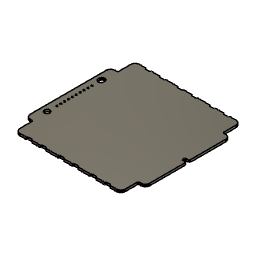
usrr5 board v2 (Autodesk Fusion 360 design; units mm, degrees)
Autodesk Fusion 360 part; units mm, degrees
sketch "Sketch1" plane through (0, 0, 0) normal (0, 1, 0) x (1, 0, 0)
  line L0 (44.246, 27.952) -> (40.2487, 27.952)
  line L1 (40.2487, 27.952) -> (40.2231, 27.9018)
  line L2 (40.2231, 27.9018) -> (40.1976, 27.8251)
  line L3 (40.1976, 27.8251) -> (40.1976, 27.774)
  line L4 (40.1976, 27.774) -> (40.1465, 27.7229)
  line L5 (40.1465, 27.7229) -> (40.1209, 27.6471)
  line L6 (40.1209, 27.6471) -> (40.0707, 27.6216)
  line L7 (40.0707, 27.6216) -> (40.0452, 27.5705)
  line L8 (40.0452, 27.5705) -> (39.9941, 27.5449)
  line L9 (39.9941, 27.5449) -> (39.9174, 27.4938)
  line L10 (39.9174, 27.4938) -> (39.8663, 27.4938)
  line L11 (39.8663, 27.4938) -> (39.7905, 27.4683)
  line L12 (39.7905, 27.4683) -> (38.1861, 27.4683)
  line L13 (38.1861, 27.4683) -> (38.1095, 27.4938)
  line L14 (38.1095, 27.4938) -> (38.0593, 27.4938)
  line L15 (38.0593, 27.4938) -> (38.0082, 27.5449)
  line L16 (38.0082, 27.5449) -> (37.9315, 27.5705)
  line L17 (37.9315, 27.5705) -> (37.906, 27.6216)
  line L18 (37.906, 27.6216) -> (37.8549, 27.6471)
  line L19 (37.8549, 27.6471) -> (37.8302, 27.6974)
  line L20 (37.8302, 27.6974) -> (37.7791, 27.774)
  line L21 (37.7791, 27.774) -> (37.7791, 27.8251)
  line L22 (37.7791, 27.8251) -> (37.7535, 27.9018)
  line L23 (37.7535, 27.9018) -> (37.728, 27.952)
  line L24 (37.728, 27.952) -> (31.9738, 27.952)
  line L25 (31.9738, 27.952) -> (31.9738, 27.9018)
  line L26 (31.9738, 27.9018) -> (31.9483, 27.8251)
  line L27 (31.9483, 27.8251) -> (31.9483, 27.774)
  line L28 (31.9483, 27.774) -> (31.8972, 27.7229)
  line L29 (31.8972, 27.7229) -> (31.8716, 27.6471)
  line L30 (31.8716, 27.6471) -> (31.8205, 27.6216)
  line L31 (31.8205, 27.6216) -> (31.7959, 27.5705)
  line L32 (31.7959, 27.5705) -> (31.7448, 27.5449)
  line L33 (31.7448, 27.5449) -> (31.6681, 27.4938)
  line L34 (31.6681, 27.4938) -> (31.617, 27.4938)
  line L35 (31.617, 27.4938) -> (31.5412, 27.4683)
  line L36 (31.5412, 27.4683) -> (29.9368, 27.4683)
  line L37 (29.9368, 27.4683) -> (29.8602, 27.4938)
  line L38 (29.8602, 27.4938) -> (29.8091, 27.4938)
  line L39 (29.8091, 27.4938) -> (29.7589, 27.5449)
  line L40 (29.7589, 27.5449) -> (29.6822, 27.5705)
  line L41 (29.6822, 27.5705) -> (29.6567, 27.6216)
  line L42 (29.6567, 27.6216) -> (29.6056, 27.6471)
  line L43 (29.6056, 27.6471) -> (29.58, 27.6974)
  line L44 (29.58, 27.6974) -> (29.5298, 27.774)
  line L45 (29.5298, 27.774) -> (29.5298, 27.8251)
  line L46 (29.5298, 27.8251) -> (29.5042, 27.9018)
  line L47 (29.5042, 27.9018) -> (29.4787, 27.952)
  line L48 (29.4787, 27.952) -> (25.4814, 27.952)
  line L49 (25.4814, 27.952) -> (25.4558, 27.9018)
  line L50 (25.4558, 27.9018) -> (25.4303, 27.8251)
  line L51 (25.4303, 27.8251) -> (25.4303, 27.774)
  line L52 (25.4303, 27.774) -> (25.3792, 27.7229)
  line L53 (25.3792, 27.7229) -> (25.3536, 27.6471)
  line L54 (25.3536, 27.6471) -> (25.3025, 27.6216)
  line L55 (25.3025, 27.6216) -> (25.2778, 27.5705)
  line L56 (25.2778, 27.5705) -> (25.2267, 27.5449)
  line L57 (25.2267, 27.5449) -> (25.1501, 27.4938)
  line L58 (25.1501, 27.4938) -> (25.099, 27.4938)
  line L59 (25.099, 27.4938) -> (25.0232, 27.4683)
  line L60 (25.0232, 27.4683) -> (23.4188, 27.4683)
  line L61 (23.4188, 27.4683) -> (23.3422, 27.4938)
  line L62 (23.3422, 27.4938) -> (23.2911, 27.4938)
  line L63 (23.2911, 27.4938) -> (23.2408, 27.5449)
  line L64 (23.2408, 27.5449) -> (23.1642, 27.5705)
  line L65 (23.1642, 27.5705) -> (23.1386, 27.6216)
  line L66 (23.1386, 27.6216) -> (23.0875, 27.6471)
  line L67 (23.0875, 27.6471) -> (23.062, 27.6974)
  line L68 (23.062, 27.6974) -> (23.0118, 27.774)
  line L69 (23.0118, 27.774) -> (23.0118, 27.8251)
  line L70 (23.0118, 27.8251) -> (22.9862, 27.9018)
  line L71 (22.9862, 27.9018) -> (22.9862, 27.952)
  line L72 (22.9862, 27.952) -> (17.2321, 27.952)
  line L73 (17.2321, 27.952) -> (17.2065, 27.9018)
  line L74 (17.2065, 27.9018) -> (17.181, 27.8251)
  line L75 (17.181, 27.8251) -> (17.181, 27.774)
  line L76 (17.181, 27.774) -> (17.1299, 27.7229)
  line L77 (17.1299, 27.7229) -> (17.1043, 27.6471)
  line L78 (17.1043, 27.6471) -> (17.0532, 27.6216)
  line L79 (17.0532, 27.6216) -> (17.0276, 27.5705)
  line L80 (17.0276, 27.5705) -> (16.9774, 27.5449)
  line L81 (16.9774, 27.5449) -> (16.9008, 27.4938)
  line L82 (16.9008, 27.4938) -> (16.8497, 27.4938)
  line L83 (16.8497, 27.4938) -> (16.773, 27.4683)
  line L84 (16.773, 27.4683) -> (15.1695, 27.4683)
  line L85 (15.1695, 27.4683) -> (15.0929, 27.4938)
  line L86 (15.0929, 27.4938) -> (15.0418, 27.4938)
  line L87 (15.0418, 27.4938) -> (14.9915, 27.5449)
  line L88 (14.9915, 27.5449) -> (14.9149, 27.5705)
  line L89 (14.9149, 27.5705) -> (14.8893, 27.6216)
  line L90 (14.8893, 27.6216) -> (14.8382, 27.6471)
  line L91 (14.8382, 27.6471) -> (14.8127, 27.6974)
  line L92 (14.8127, 27.6974) -> (14.7616, 27.774)
  line L93 (14.7616, 27.774) -> (14.7616, 27.8251)
  line L94 (14.7616, 27.8251) -> (14.7369, 27.9018)
  line L95 (14.7369, 27.9018) -> (14.7114, 27.952)
  line L96 (14.7114, 27.952) -> (10.714, 27.952)
  line L97 (10.714, 27.952) -> (10.6885, 27.9018)
  line L98 (10.6885, 27.9018) -> (10.6629, 27.8251)
  line L99 (10.6629, 27.8251) -> (10.6629, 27.774)
  line L100 (10.6629, 27.774) -> (10.6118, 27.7229)
  line L101 (10.6118, 27.7229) -> (10.5863, 27.6471)
  line L102 (10.5863, 27.6471) -> (10.5352, 27.6216)
  line L103 (10.5352, 27.6216) -> (10.5096, 27.5705)
  line L104 (10.5096, 27.5705) -> (10.4594, 27.5449)
  line L105 (10.4594, 27.5449) -> (10.3827, 27.4938)
  line L106 (10.3827, 27.4938) -> (10.3316, 27.4938)
  line L107 (10.3316, 27.4938) -> (10.255, 27.4683)
  line L108 (10.255, 27.4683) -> (8.6515, 27.4683)
  line L109 (8.6515, 27.4683) -> (8.5748, 27.4938)
  line L110 (8.5748, 27.4938) -> (8.5237, 27.4938)
  line L111 (8.5237, 27.4938) -> (8.4735, 27.5449)
  line L112 (8.4735, 27.5449) -> (8.3969, 27.5705)
  line L113 (8.3969, 27.5705) -> (8.3713, 27.6216)
  line L114 (8.3713, 27.6216) -> (8.3202, 27.6471)
  line L115 (8.3202, 27.6471) -> (8.2946, 27.6974)
  line L116 (8.2946, 27.6974) -> (8.2435, 27.774)
  line L117 (8.2435, 27.774) -> (8.2435, 27.8251)
  line L118 (8.2435, 27.8251) -> (8.2189, 27.9018)
  line L119 (8.2189, 27.9018) -> (8.2189, 27.952)
  line L120 (8.2189, 27.952) -> (5.2647, 27.952)
  line L121 (5.2647, 27.952) -> (5.0101, 27.9264)
  line L122 (5.0101, 27.9264) -> (4.7555, 27.8762)
  line L123 (4.7555, 27.8762) -> (4.5008, 27.7996)
  line L124 (4.5008, 27.7996) -> (4.2718, 27.6974)
  line L125 (4.2718, 27.6974) -> (4.0682, 27.5449)
  line L126 (4.0682, 27.5449) -> (3.8647, 27.367)
  line L127 (3.8647, 27.367) -> (3.6867, 27.1626)
  line L128 (3.6867, 27.1626) -> (3.5334, 26.959)
  line L129 (3.5334, 26.959) -> (3.4321, 26.73)
  line L130 (3.4321, 26.73) -> (3.3555, 26.4753)
  line L131 (3.3555, 26.4753) -> (3.2533, 25.9661)
  line L132 (3.2533, 25.9661) -> (3.2533, 20.4155)
  line L133 (3.2533, 20.4155) -> (3.2277, 20.3397)
  line L134 (3.2277, 20.3397) -> (3.2277, 20.2886)
  line L135 (3.2277, 20.2886) -> (3.1775, 20.2375)
  line L136 (3.1775, 20.2375) -> (3.1519, 20.1608)
  line L137 (3.1519, 20.1608) -> (3.1008, 20.1362)
  line L138 (3.1008, 20.1362) -> (3.0753, 20.0851)
  line L139 (3.0753, 20.0851) -> (3.0242, 20.0595)
  line L140 (3.0242, 20.0595) -> (2.9484, 20.0084)
  line L141 (2.9484, 20.0084) -> (2.8973, 20.0084)
  line L142 (2.8973, 20.0084) -> (2.8207, 19.9829)
  line L143 (2.8207, 19.9829) -> (2.7696, 19.9573)
  line L144 (2.7696, 19.9573) -> (1.9555, 19.9573)
  line L145 (1.9555, 19.9573) -> (1.7008, 19.9062)
  line L146 (1.7008, 19.9062) -> (1.4462, 19.856)
  line L147 (1.4462, 19.856) -> (1.1916, 19.7793)
  line L148 (1.1916, 19.7793) -> (0.9616, 19.6771)
  line L149 (0.9616, 19.6771) -> (0.7581, 19.5247)
  line L150 (0.7581, 19.5247) -> (0.5546, 19.3467)
  line L151 (0.5546, 19.3467) -> (0.3766, 19.1423)
  line L152 (0.3766, 19.1423) -> (0.2233, 18.9388)
  line L153 (0.2233, 18.9388) -> (0.122, 18.7097)
  line L154 (0.122, 18.7097) -> (0.0453, 18.4551)
  line L155 (0.0453, 18.4551) -> (-0.0058, 18.2005)
  line L156 (-0.0058, 18.2005) -> (-0.0313, 17.9459)
  line L157 (-0.0313, 17.9459) -> (-0.0313, -17.0628)
  line L158 (-0.0313, -17.0628) -> (-0.0058, -17.3174)
  line L159 (-0.0058, -17.3174) -> (0.0453, -17.572)
  line L160 (0.0453, -17.572) -> (0.122, -17.8267)
  line L161 (0.122, -17.8267) -> (0.2233, -18.0557)
  line L162 (0.2233, -18.0557) -> (0.3766, -18.2593)
  line L163 (0.3766, -18.2593) -> (0.5546, -18.4637)
  line L164 (0.5546, -18.4637) -> (0.7581, -18.6416)
  line L165 (0.7581, -18.6416) -> (0.9616, -18.7941)
  line L166 (0.9616, -18.7941) -> (1.1916, -18.8963)
  line L167 (1.1916, -18.8963) -> (1.4462, -18.9729)
  line L168 (1.4462, -18.9729) -> (1.7008, -19.0231)
  line L169 (1.7008, -19.0231) -> (1.9555, -19.0742)
  line L170 (1.9555, -19.0742) -> (2.7696, -19.0742)
  line L171 (2.7696, -19.0742) -> (2.8207, -19.0998)
  line L172 (2.8207, -19.0998) -> (2.8973, -19.1253)
  line L173 (2.8973, -19.1253) -> (2.9484, -19.1253)
  line L174 (2.9484, -19.1253) -> (2.9986, -19.1764)
  line L175 (2.9986, -19.1764) -> (3.0753, -19.202)
  line L176 (3.0753, -19.202) -> (3.1008, -19.2522)
  line L177 (3.1008, -19.2522) -> (3.1519, -19.2778)
  line L178 (3.1519, -19.2778) -> (3.1775, -19.3289)
  line L179 (3.1775, -19.3289) -> (3.2277, -19.4055)
  line L180 (3.2277, -19.4055) -> (3.2277, -19.4566)
  line L181 (3.2277, -19.4566) -> (3.2533, -19.5324)
  line L182 (3.2533, -19.5324) -> (3.2533, -25.083)
  line L183 (3.2533, -25.083) -> (3.3555, -25.5923)
  line L184 (3.3555, -25.5923) -> (3.4321, -25.8469)
  line L185 (3.4321, -25.8469) -> (3.5334, -26.076)
  line L186 (3.5334, -26.076) -> (3.6867, -26.2795)
  line L187 (3.6867, -26.2795) -> (3.8647, -26.4839)
  line L188 (3.8647, -26.4839) -> (4.0682, -26.6619)
  line L189 (4.0682, -26.6619) -> (4.2718, -26.8143)
  line L190 (4.2718, -26.8143) -> (4.5008, -26.9165)
  line L191 (4.5008, -26.9165) -> (4.7555, -26.9931)
  line L192 (4.7555, -26.9931) -> (5.0101, -27.0434)
  line L193 (5.0101, -27.0434) -> (5.2647, -27.0689)
  line L194 (5.2647, -27.0689) -> (8.2189, -27.0689)
  line L195 (8.2189, -27.0689) -> (8.2189, -27.0187)
  line L196 (8.2189, -27.0187) -> (8.2435, -26.942)
  line L197 (8.2435, -26.942) -> (8.2435, -26.8909)
  line L198 (8.2435, -26.8909) -> (8.2946, -26.8398)
  line L199 (8.2946, -26.8398) -> (8.3202, -26.7641)
  line L200 (8.3202, -26.7641) -> (8.3713, -26.7385)
  line L201 (8.3713, -26.7385) -> (8.3969, -26.6874)
  line L202 (8.3969, -26.6874) -> (8.448, -26.6619)
  line L203 (8.448, -26.6619) -> (8.5237, -26.6108)
  line L204 (8.5237, -26.6108) -> (8.5748, -26.6108)
  line L205 (8.5748, -26.6108) -> (8.6515, -26.5852)
  line L206 (8.6515, -26.5852) -> (10.255, -26.5852)
  line L207 (10.255, -26.5852) -> (10.3316, -26.6108)
  line L208 (10.3316, -26.6108) -> (10.3827, -26.6108)
  line L209 (10.3827, -26.6108) -> (10.4338, -26.6619)
  line L210 (10.4338, -26.6619) -> (10.5096, -26.6874)
  line L211 (10.5096, -26.6874) -> (10.5352, -26.7385)
  line L212 (10.5352, -26.7385) -> (10.5863, -26.7641)
  line L213 (10.5863, -26.7641) -> (10.6118, -26.8143)
  line L214 (10.6118, -26.8143) -> (10.6629, -26.8909)
  line L215 (10.6629, -26.8909) -> (10.6629, -26.942)
  line L216 (10.6629, -26.942) -> (10.6885, -27.0187)
  line L217 (10.6885, -27.0187) -> (10.714, -27.0689)
  line L218 (10.714, -27.0689) -> (14.7114, -27.0689)
  line L219 (14.7114, -27.0689) -> (14.7369, -27.0187)
  line L220 (14.7369, -27.0187) -> (14.7616, -26.942)
  line L221 (14.7616, -26.942) -> (14.7616, -26.8909)
  line L222 (14.7616, -26.8909) -> (14.8127, -26.8398)
  line L223 (14.8127, -26.8398) -> (14.8382, -26.7641)
  line L224 (14.8382, -26.7641) -> (14.8893, -26.7385)
  line L225 (14.8893, -26.7385) -> (14.9149, -26.6874)
  line L226 (14.9149, -26.6874) -> (14.966, -26.6619)
  line L227 (14.966, -26.6619) -> (15.0418, -26.6108)
  line L228 (15.0418, -26.6108) -> (15.0929, -26.6108)
  line L229 (15.0929, -26.6108) -> (15.1695, -26.5852)
  line L230 (15.1695, -26.5852) -> (16.773, -26.5852)
  line L231 (16.773, -26.5852) -> (16.8497, -26.6108)
  line L232 (16.8497, -26.6108) -> (16.9008, -26.6108)
  line L233 (16.9008, -26.6108) -> (16.9519, -26.6619)
  line L234 (16.9519, -26.6619) -> (17.0276, -26.6874)
  line L235 (17.0276, -26.6874) -> (17.0532, -26.7385)
  line L236 (17.0532, -26.7385) -> (17.1043, -26.7641)
  line L237 (17.1043, -26.7641) -> (17.1299, -26.8143)
  line L238 (17.1299, -26.8143) -> (17.181, -26.8909)
  line L239 (17.181, -26.8909) -> (17.181, -26.942)
  line L240 (17.181, -26.942) -> (17.2065, -27.0187)
  line L241 (17.2065, -27.0187) -> (17.2321, -27.0689)
  line L242 (17.2321, -27.0689) -> (22.9862, -27.0689)
  line L243 (22.9862, -27.0689) -> (22.9862, -27.0187)
  line L244 (22.9862, -27.0187) -> (23.0118, -26.942)
  line L245 (23.0118, -26.942) -> (23.0118, -26.8909)
  line L246 (23.0118, -26.8909) -> (23.062, -26.8398)
  line L247 (23.062, -26.8398) -> (23.0875, -26.7641)
  line L248 (23.0875, -26.7641) -> (23.1386, -26.7385)
  line L249 (23.1386, -26.7385) -> (23.1642, -26.6874)
  line L250 (23.1642, -26.6874) -> (23.2153, -26.6619)
  line L251 (23.2153, -26.6619) -> (23.2911, -26.6108)
  line L252 (23.2911, -26.6108) -> (23.3422, -26.6108)
  line L253 (23.3422, -26.6108) -> (23.4188, -26.5852)
  line L254 (23.4188, -26.5852) -> (25.0232, -26.5852)
  line L255 (25.0232, -26.5852) -> (25.099, -26.6108)
  line L256 (25.099, -26.6108) -> (25.1501, -26.6108)
  line L257 (25.1501, -26.6108) -> (25.2012, -26.6619)
  line L258 (25.2012, -26.6619) -> (25.2778, -26.6874)
  line L259 (25.2778, -26.6874) -> (25.3025, -26.7385)
  line L260 (25.3025, -26.7385) -> (25.3536, -26.7641)
  line L261 (25.3536, -26.7641) -> (25.3792, -26.8143)
  line L262 (25.3792, -26.8143) -> (25.4303, -26.8909)
  line L263 (25.4303, -26.8909) -> (25.4303, -26.942)
  line L264 (25.4303, -26.942) -> (25.4558, -27.0187)
  line L265 (25.4558, -27.0187) -> (25.4814, -27.0689)
  line L266 (25.4814, -27.0689) -> (29.4787, -27.0689)
  line L267 (29.4787, -27.0689) -> (29.5042, -27.0187)
  line L268 (29.5042, -27.0187) -> (29.5298, -26.942)
  line L269 (29.5298, -26.942) -> (29.5298, -26.8909)
  line L270 (29.5298, -26.8909) -> (29.58, -26.8398)
  line L271 (29.58, -26.8398) -> (29.6056, -26.7641)
  line L272 (29.6056, -26.7641) -> (29.6567, -26.7385)
  line L273 (29.6567, -26.7385) -> (29.6822, -26.6874)
  line L274 (29.6822, -26.6874) -> (29.7333, -26.6619)
  line L275 (29.7333, -26.6619) -> (29.8091, -26.6108)
  line L276 (29.8091, -26.6108) -> (29.8602, -26.6108)
  line L277 (29.8602, -26.6108) -> (29.9368, -26.5852)
  line L278 (29.9368, -26.5852) -> (31.5412, -26.5852)
  line L279 (31.5412, -26.5852) -> (31.617, -26.6108)
  line L280 (31.617, -26.6108) -> (31.6681, -26.6108)
  line L281 (31.6681, -26.6108) -> (31.7192, -26.6619)
  line L282 (31.7192, -26.6619) -> (31.7959, -26.6874)
  line L283 (31.7959, -26.6874) -> (31.8205, -26.7385)
  line L284 (31.8205, -26.7385) -> (31.8716, -26.7641)
  line L285 (31.8716, -26.7641) -> (31.8972, -26.8143)
  line L286 (31.8972, -26.8143) -> (31.9483, -26.8909)
  line L287 (31.9483, -26.8909) -> (31.9483, -26.942)
  line L288 (31.9483, -26.942) -> (31.9738, -27.0187)
  line L289 (31.9738, -27.0187) -> (31.9738, -27.0689)
  line L290 (31.9738, -27.0689) -> (37.7535, -27.0689)
  line L291 (37.7535, -27.0689) -> (37.7535, -27.0187)
  line L292 (37.7535, -27.0187) -> (37.7791, -26.942)
  line L293 (37.7791, -26.942) -> (37.7791, -26.8909)
  line L294 (37.7791, -26.8909) -> (37.8302, -26.8398)
  line L295 (37.8302, -26.8398) -> (37.8549, -26.7641)
  line L296 (37.8549, -26.7641) -> (37.906, -26.7385)
  line L297 (37.906, -26.7385) -> (37.9315, -26.6874)
  line L298 (37.9315, -26.6874) -> (37.9826, -26.6619)
  line L299 (37.9826, -26.6619) -> (38.0593, -26.6108)
  line L300 (38.0593, -26.6108) -> (38.1095, -26.6108)
  line L301 (38.1095, -26.6108) -> (38.1861, -26.5852)
  line L302 (38.1861, -26.5852) -> (39.7905, -26.5852)
  line L303 (39.7905, -26.5852) -> (39.8663, -26.6108)
  line L304 (39.8663, -26.6108) -> (39.9174, -26.6108)
  line L305 (39.9174, -26.6108) -> (39.9685, -26.6619)
  line L306 (39.9685, -26.6619) -> (40.0452, -26.6874)
  line L307 (40.0452, -26.6874) -> (40.0707, -26.7385)
  line L308 (40.0707, -26.7385) -> (40.1209, -26.7641)
  line L309 (40.1209, -26.7641) -> (40.1465, -26.8143)
  line L310 (40.1465, -26.8143) -> (40.1976, -26.8909)
  line L311 (40.1976, -26.8909) -> (40.1976, -26.942)
  line L312 (40.1976, -26.942) -> (40.2231, -27.0187)
  line L313 (40.2231, -27.0187) -> (40.2487, -27.0689)
  line L314 (40.2487, -27.0689) -> (44.246, -27.0689)
  line L315 (44.246, -27.0689) -> (44.2716, -27.0187)
  line L316 (44.2716, -27.0187) -> (44.2971, -26.942)
  line L317 (44.2971, -26.942) -> (44.2971, -26.8909)
  line L318 (44.2971, -26.8909) -> (44.3482, -26.8398)
  line L319 (44.3482, -26.8398) -> (44.3729, -26.7641)
  line L320 (44.3729, -26.7641) -> (44.424, -26.7385)
  line L321 (44.424, -26.7385) -> (44.4496, -26.6874)
  line L322 (44.4496, -26.6874) -> (44.5007, -26.6619)
  line L323 (44.5007, -26.6619) -> (44.5773, -26.6108)
  line L324 (44.5773, -26.6108) -> (44.6275, -26.6108)
  line L325 (44.6275, -26.6108) -> (44.7042, -26.5852)
  line L326 (44.7042, -26.5852) -> (46.3086, -26.5852)
  line L327 (46.3086, -26.5852) -> (46.3843, -26.6108)
  line L328 (46.3843, -26.6108) -> (46.4354, -26.6108)
  line L329 (46.4354, -26.6108) -> (46.4865, -26.6619)
  line L330 (46.4865, -26.6619) -> (46.5632, -26.6874)
  line L331 (46.5632, -26.6874) -> (46.5887, -26.7385)
  line L332 (46.5887, -26.7385) -> (46.639, -26.7641)
  line L333 (46.639, -26.7641) -> (46.6645, -26.8143)
  line L334 (46.6645, -26.8143) -> (46.7156, -26.8909)
  line L335 (46.7156, -26.8909) -> (46.7156, -26.942)
  line L336 (46.7156, -26.942) -> (46.7412, -27.0187)
  line L337 (46.7412, -27.0187) -> (46.7412, -27.0689)
  line L338 (46.7412, -27.0689) -> (49.6945, -27.0689)
  line L339 (49.6945, -27.0689) -> (49.9491, -27.0434)
  line L340 (49.9491, -27.0434) -> (50.2037, -26.9931)
  line L341 (50.2037, -26.9931) -> (50.4583, -26.9165)
  line L342 (50.4583, -26.9165) -> (50.6874, -26.8143)
  line L343 (50.6874, -26.8143) -> (50.8909, -26.6619)
  line L344 (50.8909, -26.6619) -> (51.0953, -26.4839)
  line L345 (51.0953, -26.4839) -> (51.2733, -26.2795)
  line L346 (51.2733, -26.2795) -> (51.4257, -26.076)
  line L347 (51.4257, -26.076) -> (51.5279, -25.8469)
  line L348 (51.5279, -25.8469) -> (51.6046, -25.5923)
  line L349 (51.6046, -25.5923) -> (51.6548, -25.3376)
  line L350 (51.6548, -25.3376) -> (51.7059, -25.083)
  line L351 (51.7059, -25.083) -> (51.7059, -19.5324)
  line L352 (51.7059, -19.5324) -> (51.7315, -19.4566)
  line L353 (51.7315, -19.4566) -> (51.7315, -19.4055)
  line L354 (51.7315, -19.4055) -> (51.7826, -19.3544)
  line L355 (51.7826, -19.3544) -> (51.8081, -19.2778)
  line L356 (51.8081, -19.2778) -> (51.8592, -19.2522)
  line L357 (51.8592, -19.2522) -> (51.8848, -19.202)
  line L358 (51.8848, -19.202) -> (51.935, -19.1764)
  line L359 (51.935, -19.1764) -> (52.0116, -19.1253)
  line L360 (52.0116, -19.1253) -> (52.0627, -19.1253)
  line L361 (52.0627, -19.1253) -> (52.1385, -19.0998)
  line L362 (52.1385, -19.0998) -> (52.1896, -19.0742)
  line L363 (52.1896, -19.0742) -> (53.0046, -19.0742)
  line L364 (53.0046, -19.0742) -> (53.2592, -19.0231)
  line L365 (53.2592, -19.0231) -> (53.5138, -18.9729)
  line L366 (53.5138, -18.9729) -> (53.7685, -18.8963)
  line L367 (53.7685, -18.8963) -> (53.9975, -18.7941)
  line L368 (53.9975, -18.7941) -> (54.201, -18.6416)
  line L369 (54.201, -18.6416) -> (54.4046, -18.4637)
  line L370 (54.4046, -18.4637) -> (54.5834, -18.2593)
  line L371 (54.5834, -18.2593) -> (54.7359, -18.0557)
  line L372 (54.7359, -18.0557) -> (54.8381, -17.8267)
  line L373 (54.8381, -17.8267) -> (54.9138, -17.572)
  line L374 (54.9138, -17.572) -> (54.9649, -17.3174)
  line L375 (54.9649, -17.3174) -> (54.9905, -17.0628)
  line L376 (54.9905, -17.0628) -> (54.9905, -0.7677)
  line L377 (54.9905, -0.7677) -> (54.9649, -0.6911)
  line L378 (54.9649, -0.6911) -> (54.9649, -0.6408)
  line L379 (54.9649, -0.6408) -> (54.9138, -0.5642)
  line L380 (54.9138, -0.5642) -> (54.8892, -0.5131)
  line L381 (54.8892, -0.5131) -> (54.8381, -0.4875)
  line L382 (54.8381, -0.4875) -> (54.8125, -0.4364)
  line L383 (54.8125, -0.4364) -> (54.7359, -0.4118)
  line L384 (54.7359, -0.4118) -> (54.6847, -0.3607)
  line L385 (54.6847, -0.3607) -> (54.6345, -0.3607)
  line L386 (54.6345, -0.3607) -> (54.5579, -0.3351)
  line L387 (54.5579, -0.3351) -> (54.5068, -0.3096)
  line L388 (54.5068, -0.3096) -> (53.5138, -0.3096)
  line L389 (53.5138, -0.3096) -> (53.4627, -0.284)
  line L390 (53.4627, -0.284) -> (53.387, -0.2585)
  line L391 (53.387, -0.2585) -> (53.3359, -0.2585)
  line L392 (53.3359, -0.2585) -> (53.2848, -0.2074)
  line L393 (53.2848, -0.2074) -> (53.2081, -0.1827)
  line L394 (53.2081, -0.1827) -> (53.1826, -0.1316)
  line L395 (53.1826, -0.1316) -> (53.1323, -0.106)
  line L396 (53.1323, -0.106) -> (53.1068, -0.0549)
  line L397 (53.1068, -0.0549) -> (53.0557, 0.0217)
  line L398 (53.0557, 0.0217) -> (53.0557, 0.0719)
  line L399 (53.0557, 0.0719) -> (53.0301, 0.1486)
  line L400 (53.0301, 0.1486) -> (53.0046, 0.1997)
  line L401 (53.0046, 0.1997) -> (53.0046, 0.6834)
  line L402 (53.0046, 0.6834) -> (53.0301, 0.7345)
  line L403 (53.0301, 0.7345) -> (53.0557, 0.8111)
  line L404 (53.0557, 0.8111) -> (53.0557, 0.8614)
  line L405 (53.0557, 0.8614) -> (53.1068, 0.9125)
  line L406 (53.1068, 0.9125) -> (53.1323, 0.9891)
  line L407 (53.1323, 0.9891) -> (53.1826, 1.0147)
  line L408 (53.1826, 1.0147) -> (53.2081, 1.0658)
  line L409 (53.2081, 1.0658) -> (53.2592, 1.0904)
  line L410 (53.2592, 1.0904) -> (53.3359, 1.1415)
  line L411 (53.3359, 1.1415) -> (53.387, 1.1415)
  line L412 (53.387, 1.1415) -> (53.4627, 1.1671)
  line L413 (53.4627, 1.1671) -> (53.5138, 1.1926)
  line L414 (53.5138, 1.1926) -> (54.5068, 1.1926)
  line L415 (54.5068, 1.1926) -> (54.5579, 1.2182)
  line L416 (54.5579, 1.2182) -> (54.6345, 1.2437)
  line L417 (54.6345, 1.2437) -> (54.6847, 1.2437)
  line L418 (54.6847, 1.2437) -> (54.7614, 1.2948)
  line L419 (54.7614, 1.2948) -> (54.8125, 1.3204)
  line L420 (54.8125, 1.3204) -> (54.8381, 1.3706)
  line L421 (54.8381, 1.3706) -> (54.8892, 1.3962)
  line L422 (54.8892, 1.3962) -> (54.9138, 1.4728)
  line L423 (54.9138, 1.4728) -> (54.9649, 1.5239)
  line L424 (54.9649, 1.5239) -> (54.9649, 1.5741)
  line L425 (54.9649, 1.5741) -> (54.9905, 1.6508)
  line L426 (54.9905, 1.6508) -> (54.9905, 17.9459)
  line L427 (54.9905, 17.9459) -> (54.9649, 18.2005)
  line L428 (54.9649, 18.2005) -> (54.9138, 18.4551)
  line L429 (54.9138, 18.4551) -> (54.8381, 18.7097)
  line L430 (54.8381, 18.7097) -> (54.7359, 18.9388)
  line L431 (54.7359, 18.9388) -> (54.5834, 19.1423)
  line L432 (54.5834, 19.1423) -> (54.4046, 19.3467)
  line L433 (54.4046, 19.3467) -> (54.201, 19.5247)
  line L434 (54.201, 19.5247) -> (53.9975, 19.6771)
  line L435 (53.9975, 19.6771) -> (53.7685, 19.7793)
  line L436 (53.7685, 19.7793) -> (53.5138, 19.856)
  line L437 (53.5138, 19.856) -> (53.2592, 19.9062)
  line L438 (53.2592, 19.9062) -> (53.0046, 19.9573)
  line L439 (53.0046, 19.9573) -> (52.1896, 19.9573)
  line L440 (52.1896, 19.9573) -> (52.1385, 19.9829)
  line L441 (52.1385, 19.9829) -> (52.0627, 20.0084)
  line L442 (52.0627, 20.0084) -> (52.0116, 20.0084)
  line L443 (52.0116, 20.0084) -> (51.9605, 20.0595)
  line L444 (51.9605, 20.0595) -> (51.8848, 20.0851)
  line L445 (51.8848, 20.0851) -> (51.8592, 20.1362)
  line L446 (51.8592, 20.1362) -> (51.8081, 20.1608)
  line L447 (51.8081, 20.1608) -> (51.7826, 20.2119)
  line L448 (51.7826, 20.2119) -> (51.7315, 20.2886)
  line L449 (51.7315, 20.2886) -> (51.7315, 20.3397)
  line L450 (51.7315, 20.3397) -> (51.7059, 20.4155)
  line L451 (51.7059, 20.4155) -> (51.7059, 25.9661)
  line L452 (51.7059, 25.9661) -> (51.6548, 26.2207)
  line L453 (51.6548, 26.2207) -> (51.6046, 26.4753)
  line L454 (51.6046, 26.4753) -> (51.5279, 26.73)
  line L455 (51.5279, 26.73) -> (51.4257, 26.959)
  line L456 (51.4257, 26.959) -> (51.2733, 27.1626)
  line L457 (51.2733, 27.1626) -> (51.0953, 27.367)
  line L458 (51.0953, 27.367) -> (50.8909, 27.5449)
  line L459 (50.8909, 27.5449) -> (50.6874, 27.6974)
  line L460 (50.6874, 27.6974) -> (50.4583, 27.7996)
  line L461 (50.4583, 27.7996) -> (50.2037, 27.8762)
  line L462 (50.2037, 27.8762) -> (49.9491, 27.9264)
  line L463 (49.9491, 27.9264) -> (49.6945, 27.952)
  line L464 (49.6945, 27.952) -> (46.7412, 27.952)
  line L465 (46.7412, 27.952) -> (46.7412, 27.9018)
  line L466 (46.7412, 27.9018) -> (46.7156, 27.8251)
  line L467 (46.7156, 27.8251) -> (46.7156, 27.774)
  line L468 (46.7156, 27.774) -> (46.6645, 27.7229)
  line L469 (46.6645, 27.7229) -> (46.639, 27.6471)
  line L470 (46.639, 27.6471) -> (46.5887, 27.6216)
  line L471 (46.5887, 27.6216) -> (46.5632, 27.5705)
  line L472 (46.5632, 27.5705) -> (46.5121, 27.5449)
  line L473 (46.5121, 27.5449) -> (46.4354, 27.4938)
  line L474 (46.4354, 27.4938) -> (46.3843, 27.4938)
  line L475 (46.3843, 27.4938) -> (46.3086, 27.4683)
  line L476 (46.3086, 27.4683) -> (44.7042, 27.4683)
  line L477 (44.7042, 27.4683) -> (44.6275, 27.4938)
  line L478 (44.6275, 27.4938) -> (44.5773, 27.4938)
  line L479 (44.5773, 27.4938) -> (44.5262, 27.5449)
  line L480 (44.5262, 27.5449) -> (44.4496, 27.5705)
  line L481 (44.4496, 27.5705) -> (44.424, 27.6216)
  line L482 (44.424, 27.6216) -> (44.3729, 27.6471)
  line L483 (44.3729, 27.6471) -> (44.3482, 27.6974)
  line L484 (44.3482, 27.6974) -> (44.2971, 27.774)
  line L485 (44.2971, 27.774) -> (44.2971, 27.8251)
  line L486 (44.2971, 27.8251) -> (44.2716, 27.9018)
  line L487 (44.2716, 27.9018) -> (44.246, 27.952)
  line L488 (1.522, 13.2102) -> (1.522, 13.3635)
  line L489 (1.522, 13.3635) -> (1.5731, 13.5415)
  line L490 (1.5731, 13.5415) -> (1.6242, 13.6939)
  line L491 (1.6242, 13.6939) -> (1.7008, 13.8216)
  line L492 (1.7008, 13.8216) -> (1.7766, 13.9741)
  line L493 (1.7766, 13.9741) -> (1.8788, 14.1018)
  line L494 (1.8788, 14.1018) -> (2.0057, 14.2031)
  line L495 (2.0057, 14.2031) -> (2.1334, 14.2798)
  line L496 (2.1334, 14.2798) -> (2.2859, 14.3564)
  line L497 (2.2859, 14.3564) -> (2.4392, 14.4067)
  line L498 (2.4392, 14.4067) -> (2.6171, 14.4578)
  line L499 (2.6171, 14.4578) -> (2.9229, 14.4578)
  line L500 (2.9229, 14.4578) -> (3.1008, 14.4067)
  line L501 (3.1008, 14.4067) -> (3.2533, 14.3564)
  line L502 (3.2533, 14.3564) -> (3.381, 14.2798)
  line L503 (3.381, 14.2798) -> (3.5334, 14.2031)
  line L504 (3.5334, 14.2031) -> (3.6612, 14.1018)
  line L505 (3.6612, 14.1018) -> (3.7625, 13.9741)
  line L506 (3.7625, 13.9741) -> (3.8392, 13.8216)
  line L507 (3.8392, 13.8216) -> (3.9158, 13.6939)
  line L508 (3.9158, 13.6939) -> (3.966, 13.5415)
  line L509 (3.966, 13.5415) -> (4.0171, 13.3635)
  line L510 (4.0171, 13.3635) -> (4.0171, 12.5485)
  line L511 (4.0171, 12.5485) -> (3.966, 12.3697)
  line L512 (3.966, 12.3697) -> (3.9158, 12.2172)
  line L513 (3.9158, 12.2172) -> (3.8392, 12.0904)
  line L514 (3.8392, 12.0904) -> (3.7625, 11.9371)
  line L515 (3.7625, 11.9371) -> (3.6612, 11.8102)
  line L516 (3.6612, 11.8102) -> (3.5334, 11.708)
  line L517 (3.5334, 11.708) -> (3.4066, 11.6313)
  line L518 (3.4066, 11.6313) -> (3.2533, 11.5556)
  line L519 (3.2533, 11.5556) -> (3.1008, 11.5045)
  line L520 (3.1008, 11.5045) -> (2.9229, 11.4534)
  line L521 (2.9229, 11.4534) -> (2.6171, 11.4534)
  line L522 (2.6171, 11.4534) -> (2.4392, 11.5045)
  line L523 (2.4392, 11.5045) -> (2.2859, 11.5556)
  line L524 (2.2859, 11.5556) -> (2.159, 11.6313)
  line L525 (2.159, 11.6313) -> (2.0057, 11.708)
  line L526 (2.0057, 11.708) -> (1.8788, 11.8102)
  line L527 (1.8788, 11.8102) -> (1.7766, 11.9371)
  line L528 (1.7766, 11.9371) -> (1.7008, 12.0904)
  line L529 (1.7008, 12.0904) -> (1.6242, 12.2172)
  line L530 (1.6242, 12.2172) -> (1.5731, 12.3697)
  line L531 (1.5731, 12.3697) -> (1.522, 12.5485)
  line L532 (1.522, 12.5485) -> (1.522, 13.2102)
  spline S0 degree 3 poles (3.9916, -12.0725) (3.9916, -12.084) (3.9916, -12.0804) (3.9916, -12.0602) knots 0 0 0 0 1 1 1 1
  spline S1 degree 3 poles (3.9916, -12.0602) (3.9916, -11.3791) (3.44, -10.8249) (2.7572, -10.8249) knots 0 0 0 0 1 1 1 1
  spline S2 degree 3 poles (2.7572, -10.8249) (2.0744, -10.8249) (1.522, -11.3791) (1.522, -12.0602) knots 0 0 0 0 1 1 1 1
  spline S3 degree 3 poles (1.522, -12.0602) (1.522, -12.7412) (2.0744, -13.2945) (2.7572, -13.2945) knots 0 0 0 0 1 1 1 1
  spline S4 degree 3 poles (2.7572, -13.2945) (3.4348, -13.2945) (3.9854, -12.7492) (3.9916, -12.0725) knots 0 0 0 0 1 1 1 1
  line L533 (3.9916, -12.0725) -> (2.7572, -12.0602)
  line L534 (2.7572, -12.0602) -> (3.9916, -12.0725)
  spline S5 degree 3 poles (3.1264, 6.745) (3.1264, 6.7459) (3.1264, 6.7494) (3.1264, 6.7556) knots 0 0 0 0 1 1 1 1
  spline S6 degree 3 poles (3.1264, 6.7556) (3.1264, 6.96) (2.9625, 7.1248) (2.7572, 7.1248) knots 0 0 0 0 1 1 1 1
  spline S7 degree 3 poles (2.7572, 7.1248) (2.5519, 7.1248) (2.3881, 6.96) (2.3881, 6.7556) knots 0 0 0 0 1 1 1 1
  spline S8 degree 3 poles (2.3881, 6.7556) (2.3881, 6.5521) (2.5519, 6.3864) (2.7572, 6.3864) knots 0 0 0 0 1 1 1 1
  spline S9 degree 3 poles (2.7572, 6.3864) (2.9564, 6.3864) (3.1202, 6.5441) (3.1264, 6.745) knots 0 0 0 0 1 1 1 1
  line L535 (3.1264, 6.745) -> (2.7572, 6.7556)
  line L536 (2.7572, 6.7556) -> (3.1264, 6.745)
  spline S10 degree 3 poles (3.1264, 4.9371) (3.1264, 4.9389) (3.1264, 4.9415) (3.1264, 4.9486) knots 0 0 0 0 1 1 1 1
  spline S11 degree 3 poles (3.1264, 4.9486) (3.1264, 5.1521) (2.9625, 5.3177) (2.7572, 5.3177) knots 0 0 0 0 1 1 1 1
  spline S12 degree 3 poles (2.7572, 5.3177) (2.5519, 5.3177) (2.3881, 5.1521) (2.3881, 4.9486) knots 0 0 0 0 1 1 1 1
  spline S13 degree 3 poles (2.3881, 4.9486) (2.3881, 4.7442) (2.5519, 4.5794) (2.7572, 4.5794) knots 0 0 0 0 1 1 1 1
  spline S14 degree 3 poles (2.7572, 4.5794) (2.9564, 4.5794) (3.1202, 4.7362) (3.1264, 4.9371) knots 0 0 0 0 1 1 1 1
  line L537 (3.1264, 4.9371) -> (2.7572, 4.9486)
  line L538 (2.7572, 4.9486) -> (3.1264, 4.9371)
  spline S15 degree 3 poles (3.1264, 3.1547) (3.1264, 3.1565) (3.1264, 3.1591) (3.1264, 3.1662) knots 0 0 0 0 1 1 1 1
  spline S16 degree 3 poles (3.1264, 3.1662) (3.1264, 3.3697) (2.9625, 3.5353) (2.7572, 3.5353) knots 0 0 0 0 1 1 1 1
  spline S17 degree 3 poles (2.7572, 3.5353) (2.5519, 3.5353) (2.3881, 3.3697) (2.3881, 3.1662) knots 0 0 0 0 1 1 1 1
  spline S18 degree 3 poles (2.3881, 3.1662) (2.3881, 2.9618) (2.5519, 2.797) (2.7572, 2.797) knots 0 0 0 0 1 1 1 1
  spline S19 degree 3 poles (2.7572, 2.797) (2.9564, 2.797) (3.1202, 2.9539) (3.1264, 3.1547) knots 0 0 0 0 1 1 1 1
  line L539 (3.1264, 3.1547) -> (2.7572, 3.1662)
  line L540 (2.7572, 3.1662) -> (3.1264, 3.1547)
  spline S20 degree 3 poles (3.1264, 1.3468) (3.1264, 1.3486) (3.1264, 1.3521) (3.1264, 1.3583) knots 0 0 0 0 1 1 1 1
  spline S21 degree 3 poles (3.1264, 1.3583) (3.1264, 1.5618) (2.9625, 1.7274) (2.7572, 1.7274) knots 0 0 0 0 1 1 1 1
  spline S22 degree 3 poles (2.7572, 1.7274) (2.5519, 1.7274) (2.3881, 1.5618) (2.3881, 1.3583) knots 0 0 0 0 1 1 1 1
  spline S23 degree 3 poles (2.3881, 1.3583) (2.3881, 1.1547) (2.5519, 0.9891) (2.7572, 0.9891) knots 0 0 0 0 1 1 1 1
  spline S24 degree 3 poles (2.7572, 0.9891) (2.9564, 0.9891) (3.1202, 1.1468) (3.1264, 1.3468) knots 0 0 0 0 1 1 1 1
  line L541 (3.1264, 1.3468) -> (2.7572, 1.3583)
  line L542 (2.7572, 1.3583) -> (3.1264, 1.3468)
  spline S25 degree 3 poles (3.1264, 8.5521) (3.1264, 8.5538) (3.1264, 8.5574) (3.1264, 8.5635) knots 0 0 0 0 1 1 1 1
  spline S26 degree 3 poles (3.1264, 8.5635) (3.1264, 8.767) (2.9625, 8.9327) (2.7572, 8.9327) knots 0 0 0 0 1 1 1 1
  spline S27 degree 3 poles (2.7572, 8.9327) (2.5519, 8.9327) (2.3881, 8.767) (2.3881, 8.5635) knots 0 0 0 0 1 1 1 1
  spline S28 degree 3 poles (2.3881, 8.5635) (2.3881, 8.36) (2.5519, 8.1944) (2.7572, 8.1944) knots 0 0 0 0 1 1 1 1
  spline S29 degree 3 poles (2.7572, 8.1944) (2.9564, 8.1944) (3.1202, 8.3521) (3.1264, 8.5521) knots 0 0 0 0 1 1 1 1
  line L543 (3.1264, 8.5521) -> (2.7572, 8.5635)
  line L544 (2.7572, 8.5635) -> (3.1264, 8.5521)
  spline S30 degree 3 poles (3.1264, -2.2682) (3.1264, -2.2673) (3.1264, -2.2637) (3.1264, -2.2576) knots 0 0 0 0 1 1 1 1
  spline S31 degree 3 poles (3.1264, -2.2576) (3.1264, -2.0541) (2.9625, -1.8884) (2.7572, -1.8884) knots 0 0 0 0 1 1 1 1
  spline S32 degree 3 poles (2.7572, -1.8884) (2.5519, -1.8884) (2.3881, -2.0541) (2.3881, -2.2576) knots 0 0 0 0 1 1 1 1
  spline S33 degree 3 poles (2.3881, -2.2576) (2.3881, -2.4611) (2.5519, -2.6267) (2.7572, -2.6267) knots 0 0 0 0 1 1 1 1
  spline S34 degree 3 poles (2.7572, -2.6267) (2.9564, -2.6267) (3.1202, -2.469) (3.1264, -2.2682) knots 0 0 0 0 1 1 1 1
  line L545 (3.1264, -2.2682) -> (2.7572, -2.2576)
  line L546 (2.7572, -2.2576) -> (3.1264, -2.2682)
  spline S35 degree 3 poles (3.1264, -4.0505) (3.1264, -4.0488) (3.1264, -4.0461) (3.1264, -4.04) knots 0 0 0 0 1 1 1 1
  spline S36 degree 3 poles (3.1264, -4.04) (3.1264, -3.8355) (2.9625, -3.6708) (2.7572, -3.6708) knots 0 0 0 0 1 1 1 1
  spline S37 degree 3 poles (2.7572, -3.6708) (2.5519, -3.6708) (2.3881, -3.8355) (2.3881, -4.04) knots 0 0 0 0 1 1 1 1
  spline S38 degree 3 poles (2.3881, -4.04) (2.3881, -4.2435) (2.5519, -4.4091) (2.7572, -4.4091) knots 0 0 0 0 1 1 1 1
  spline S39 degree 3 poles (2.7572, -4.4091) (2.9564, -4.4091) (3.1202, -4.2514) (3.1264, -4.0505) knots 0 0 0 0 1 1 1 1
  line L547 (3.1264, -4.0505) -> (2.7572, -4.04)
  line L548 (2.7572, -4.04) -> (3.1264, -4.0505)
  spline S40 degree 3 poles (3.1264, -5.8584) (3.1264, -5.8567) (3.1264, -5.854) (3.1264, -5.847) knots 0 0 0 0 1 1 1 1
  spline S41 degree 3 poles (3.1264, -5.847) (3.1264, -5.6435) (2.9625, -5.4778) (2.7572, -5.4778) knots 0 0 0 0 1 1 1 1
  spline S42 degree 3 poles (2.7572, -5.4778) (2.5519, -5.4778) (2.3881, -5.6435) (2.3881, -5.847) knots 0 0 0 0 1 1 1 1
  spline S43 degree 3 poles (2.3881, -5.847) (2.3881, -6.0514) (2.5519, -6.2162) (2.7572, -6.2162) knots 0 0 0 0 1 1 1 1
  spline S44 degree 3 poles (2.7572, -6.2162) (2.9564, -6.2162) (3.1202, -6.0593) (3.1264, -5.8584) knots 0 0 0 0 1 1 1 1
  line L549 (3.1264, -5.8584) -> (2.7572, -5.847)
  line L550 (2.7572, -5.847) -> (3.1264, -5.8584)
  spline S45 degree 3 poles (3.1264, -7.6664) (3.1264, -7.6646) (3.1264, -7.6611) (3.1264, -7.6549) knots 0 0 0 0 1 1 1 1
  spline S46 degree 3 poles (3.1264, -7.6549) (3.1264, -7.4514) (2.9625, -7.2858) (2.7572, -7.2858) knots 0 0 0 0 1 1 1 1
  spline S47 degree 3 poles (2.7572, -7.2858) (2.5519, -7.2858) (2.3881, -7.4514) (2.3881, -7.6549) knots 0 0 0 0 1 1 1 1
  spline S48 degree 3 poles (2.3881, -7.6549) (2.3881, -7.8584) (2.5519, -8.0241) (2.7572, -8.0241) knots 0 0 0 0 1 1 1 1
  spline S49 degree 3 poles (2.7572, -8.0241) (2.9564, -8.0241) (3.1202, -7.8664) (3.1264, -7.6664) knots 0 0 0 0 1 1 1 1
  line L551 (3.1264, -7.6664) -> (2.7572, -7.6549)
  line L552 (2.7572, -7.6549) -> (3.1264, -7.6664)
  spline S50 degree 3 poles (3.1264, -0.4611) (3.1264, -0.4594) (3.1264, -0.4558) (3.1264, -0.4497) knots 0 0 0 0 1 1 1 1
  spline S51 degree 3 poles (3.1264, -0.4497) (3.1264, -0.2461) (2.9625, -0.0805) (2.7572, -0.0805) knots 0 0 0 0 1 1 1 1
  spline S52 degree 3 poles (2.7572, -0.0805) (2.5519, -0.0805) (2.3881, -0.2461) (2.3881, -0.4497) knots 0 0 0 0 1 1 1 1
  spline S53 degree 3 poles (2.3881, -0.4497) (2.3881, -0.6532) (2.5519, -0.8188) (2.7572, -0.8188) knots 0 0 0 0 1 1 1 1
  spline S54 degree 3 poles (2.7572, -0.8188) (2.9564, -0.8188) (3.1202, -0.6611) (3.1264, -0.4611) knots 0 0 0 0 1 1 1 1
  line L553 (3.1264, -0.4611) -> (2.7572, -0.4497)
  line L554 (2.7572, -0.4497) -> (3.1264, -0.4611)
  line L555 (1.522, 13.2102) -> (1.522, 13.3635)
  line L556 (1.522, 13.3635) -> (1.5731, 13.5415)
  line L557 (1.5731, 13.5415) -> (1.6242, 13.6939)
  line L558 (1.6242, 13.6939) -> (1.7008, 13.8216)
  line L559 (1.7008, 13.8216) -> (1.7766, 13.9741)
  line L560 (1.7766, 13.9741) -> (1.8788, 14.1018)
  line L561 (1.8788, 14.1018) -> (2.0057, 14.2031)
  line L562 (2.0057, 14.2031) -> (2.1334, 14.2798)
  line L563 (2.1334, 14.2798) -> (2.2859, 14.3564)
  line L564 (2.2859, 14.3564) -> (2.4392, 14.4067)
  line L565 (2.4392, 14.4067) -> (2.6171, 14.4578)
  line L566 (2.6171, 14.4578) -> (2.9229, 14.4578)
  line L567 (2.9229, 14.4578) -> (3.1008, 14.4067)
  line L568 (3.1008, 14.4067) -> (3.2533, 14.3564)
  line L569 (3.2533, 14.3564) -> (3.381, 14.2798)
  line L570 (3.381, 14.2798) -> (3.5334, 14.2031)
  line L571 (3.5334, 14.2031) -> (3.6612, 14.1018)
  line L572 (3.6612, 14.1018) -> (3.7625, 13.9741)
  line L573 (3.7625, 13.9741) -> (3.8392, 13.8216)
  line L574 (3.8392, 13.8216) -> (3.9158, 13.6939)
  line L575 (3.9158, 13.6939) -> (3.966, 13.5415)
  line L576 (3.966, 13.5415) -> (4.0171, 13.3635)
  line L577 (4.0171, 13.3635) -> (4.0171, 12.5485)
  line L578 (4.0171, 12.5485) -> (3.966, 12.3697)
  line L579 (3.966, 12.3697) -> (3.9158, 12.2172)
  line L580 (3.9158, 12.2172) -> (3.8392, 12.0904)
  line L581 (3.8392, 12.0904) -> (3.7625, 11.9371)
  line L582 (3.7625, 11.9371) -> (3.6612, 11.8102)
  line L583 (3.6612, 11.8102) -> (3.5334, 11.708)
  line L584 (3.5334, 11.708) -> (3.4066, 11.6313)
  line L585 (3.4066, 11.6313) -> (3.2533, 11.5556)
  line L586 (3.2533, 11.5556) -> (3.1008, 11.5045)
  line L587 (3.1008, 11.5045) -> (2.9229, 11.4534)
  line L588 (2.9229, 11.4534) -> (2.6171, 11.4534)
  line L589 (2.6171, 11.4534) -> (2.4392, 11.5045)
  line L590 (2.4392, 11.5045) -> (2.2859, 11.5556)
  line L591 (2.2859, 11.5556) -> (2.159, 11.6313)
  line L592 (2.159, 11.6313) -> (2.0057, 11.708)
  line L593 (2.0057, 11.708) -> (1.8788, 11.8102)
  line L594 (1.8788, 11.8102) -> (1.7766, 11.9371)
  line L595 (1.7766, 11.9371) -> (1.7008, 12.0904)
  line L596 (1.7008, 12.0904) -> (1.6242, 12.2172)
  line L597 (1.6242, 12.2172) -> (1.5731, 12.3697)
  line L598 (1.5731, 12.3697) -> (1.522, 12.5485)
  line L599 (1.522, 12.5485) -> (1.522, 13.2102)
  spline S55 degree 3 poles (4.0171, -12.0981) (4.0171, -12.1016) (4.0171, -12.0937) (4.0171, -12.0725) knots 0 0 0 0 1 1 1 1
  spline S56 degree 3 poles (4.0171, -12.0725) (4.0171, -11.3853) (3.4586, -10.8249) (2.7696, -10.8249) knots 0 0 0 0 1 1 1 1
  spline S57 degree 3 poles (2.7696, -10.8249) (2.0806, -10.8249) (1.522, -11.3853) (1.522, -12.0725) knots 0 0 0 0 1 1 1 1
  spline S58 degree 3 poles (1.522, -12.0725) (1.522, -12.7597) (2.0806, -13.3201) (2.7696, -13.3201) knots 0 0 0 0 1 1 1 1
  spline S59 degree 3 poles (2.7696, -13.3201) (3.4489, -13.3201) (4.003, -12.7756) (4.0171, -12.0981) knots 0 0 0 0 1 1 1 1
  spline S60 degree 3 poles (3.1502, 6.7195) (3.1519, 6.7256) (3.1519, 6.7336) (3.1519, 6.7433) knots 0 0 0 0 1 1 1 1
  spline S61 degree 3 poles (3.1519, 6.7433) (3.1519, 6.953) (2.981, 7.1248) (2.7696, 7.1248) knots 0 0 0 0 1 1 1 1
  spline S62 degree 3 poles (2.7696, 7.1248) (2.5581, 7.1248) (2.3881, 6.953) (2.3881, 6.7433) knots 0 0 0 0 1 1 1 1
  spline S63 degree 3 poles (2.3881, 6.7433) (2.3881, 6.5327) (2.5581, 6.3609) (2.7696, 6.3609) knots 0 0 0 0 1 1 1 1
  spline S64 degree 3 poles (2.7696, 6.3609) (2.9722, 6.3609) (3.1387, 6.5186) (3.1502, 6.7195) knots 0 0 0 0 1 1 1 1
  spline S65 degree 3 poles (3.1502, 4.9116) (3.1519, 4.9177) (3.1519, 4.9256) (3.1519, 4.9353) knots 0 0 0 0 1 1 1 1
  spline S66 degree 3 poles (3.1519, 4.9353) (3.1519, 5.1459) (2.981, 5.3177) (2.7696, 5.3177) knots 0 0 0 0 1 1 1 1
  spline S67 degree 3 poles (2.7696, 5.3177) (2.5581, 5.3177) (2.3881, 5.1459) (2.3881, 4.9353) knots 0 0 0 0 1 1 1 1
  spline S68 degree 3 poles (2.3881, 4.9353) (2.3881, 4.7256) (2.5581, 4.5538) (2.7696, 4.5538) knots 0 0 0 0 1 1 1 1
  spline S69 degree 3 poles (2.7696, 4.5538) (2.9722, 4.5538) (3.1387, 4.7107) (3.1502, 4.9116) knots 0 0 0 0 1 1 1 1
  spline S70 degree 3 poles (3.1502, 3.1292) (3.1519, 3.1353) (3.1519, 3.1433) (3.1519, 3.153) knots 0 0 0 0 1 1 1 1
  spline S71 degree 3 poles (3.1519, 3.153) (3.1519, 3.3635) (2.981, 3.5353) (2.7696, 3.5353) knots 0 0 0 0 1 1 1 1
  spline S72 degree 3 poles (2.7696, 3.5353) (2.5581, 3.5353) (2.3881, 3.3635) (2.3881, 3.153) knots 0 0 0 0 1 1 1 1
  spline S73 degree 3 poles (2.3881, 3.153) (2.3881, 2.9433) (2.5581, 2.7715) (2.7696, 2.7715) knots 0 0 0 0 1 1 1 1
  spline S74 degree 3 poles (2.7696, 2.7715) (2.9722, 2.7715) (3.1387, 2.9292) (3.1502, 3.1292) knots 0 0 0 0 1 1 1 1
  spline S75 degree 3 poles (3.1502, 1.3213) (3.1519, 1.3283) (3.1519, 1.3362) (3.1519, 1.345) knots 0 0 0 0 1 1 1 1
  spline S76 degree 3 poles (3.1519, 1.345) (3.1519, 1.5556) (2.981, 1.7274) (2.7696, 1.7274) knots 0 0 0 0 1 1 1 1
  spline S77 degree 3 poles (2.7696, 1.7274) (2.5581, 1.7274) (2.3881, 1.5556) (2.3881, 1.345) knots 0 0 0 0 1 1 1 1
  spline S78 degree 3 poles (2.3881, 1.345) (2.3881, 1.1354) (2.5581, 0.9636) (2.7696, 0.9636) knots 0 0 0 0 1 1 1 1
  spline S79 degree 3 poles (2.7696, 0.9636) (2.9722, 0.9636) (3.1387, 1.1213) (3.1502, 1.3213) knots 0 0 0 0 1 1 1 1
  spline S80 degree 3 poles (3.1502, 8.5274) (3.1519, 8.5336) (3.1519, 8.5415) (3.1519, 8.5512) knots 0 0 0 0 1 1 1 1
  spline S81 degree 3 poles (3.1519, 8.5512) (3.1519, 8.7609) (2.981, 8.9327) (2.7696, 8.9327) knots 0 0 0 0 1 1 1 1
  spline S82 degree 3 poles (2.7696, 8.9327) (2.5581, 8.9327) (2.3881, 8.7609) (2.3881, 8.5512) knots 0 0 0 0 1 1 1 1
  spline S83 degree 3 poles (2.3881, 8.5512) (2.3881, 8.3406) (2.5581, 8.1688) (2.7696, 8.1688) knots 0 0 0 0 1 1 1 1
  spline S84 degree 3 poles (2.7696, 8.1688) (2.9722, 8.1688) (3.1387, 8.3265) (3.1502, 8.5274) knots 0 0 0 0 1 1 1 1
  spline S85 degree 3 poles (3.1502, -2.2937) (3.1519, -2.2875) (3.1519, -2.2796) (3.1519, -2.2699) knots 0 0 0 0 1 1 1 1
  spline S86 degree 3 poles (3.1519, -2.2699) (3.1519, -2.0602) (2.981, -1.8884) (2.7696, -1.8884) knots 0 0 0 0 1 1 1 1
  spline S87 degree 3 poles (2.7696, -1.8884) (2.5581, -1.8884) (2.3881, -2.0602) (2.3881, -2.2699) knots 0 0 0 0 1 1 1 1
  spline S88 degree 3 poles (2.3881, -2.2699) (2.3881, -2.4805) (2.5581, -2.6523) (2.7696, -2.6523) knots 0 0 0 0 1 1 1 1
  spline S89 degree 3 poles (2.7696, -2.6523) (2.9722, -2.6523) (3.1387, -2.4946) (3.1502, -2.2937) knots 0 0 0 0 1 1 1 1
  spline S90 degree 3 poles (3.1502, -4.0761) (3.1519, -4.0699) (3.1519, -4.062) (3.1519, -4.0523) knots 0 0 0 0 1 1 1 1
  spline S91 degree 3 poles (3.1519, -4.0523) (3.1519, -3.8426) (2.981, -3.6708) (2.7696, -3.6708) knots 0 0 0 0 1 1 1 1
  spline S92 degree 3 poles (2.7696, -3.6708) (2.5581, -3.6708) (2.3881, -3.8426) (2.3881, -4.0523) knots 0 0 0 0 1 1 1 1
  spline S93 degree 3 poles (2.3881, -4.0523) (2.3881, -4.262) (2.5581, -4.4347) (2.7696, -4.4347) knots 0 0 0 0 1 1 1 1
  spline S94 degree 3 poles (2.7696, -4.4347) (2.9722, -4.4347) (3.1387, -4.277) (3.1502, -4.0761) knots 0 0 0 0 1 1 1 1
  spline S95 degree 3 poles (3.1502, -5.884) (3.1519, -5.8778) (3.1519, -5.8699) (3.1519, -5.8602) knots 0 0 0 0 1 1 1 1
  spline S96 degree 3 poles (3.1519, -5.8602) (3.1519, -5.6496) (2.981, -5.4778) (2.7696, -5.4778) knots 0 0 0 0 1 1 1 1
  spline S97 degree 3 poles (2.7696, -5.4778) (2.5581, -5.4778) (2.3881, -5.6496) (2.3881, -5.8602) knots 0 0 0 0 1 1 1 1
  spline S98 degree 3 poles (2.3881, -5.8602) (2.3881, -6.0699) (2.5581, -6.2417) (2.7696, -6.2417) knots 0 0 0 0 1 1 1 1
  spline S99 degree 3 poles (2.7696, -6.2417) (2.9722, -6.2417) (3.1387, -6.0849) (3.1502, -5.884) knots 0 0 0 0 1 1 1 1
  spline S100 degree 3 poles (3.1502, -7.6919) (3.1519, -7.6858) (3.1519, -7.6778) (3.1519, -7.6681) knots 0 0 0 0 1 1 1 1
  spline S101 degree 3 poles (3.1519, -7.6681) (3.1519, -7.4576) (2.981, -7.2858) (2.7696, -7.2858) knots 0 0 0 0 1 1 1 1
  spline S102 degree 3 poles (2.7696, -7.2858) (2.5581, -7.2858) (2.3881, -7.4576) (2.3881, -7.6681) knots 0 0 0 0 1 1 1 1
  spline S103 degree 3 poles (2.3881, -7.6681) (2.3881, -7.8778) (2.5581, -8.0496) (2.7696, -8.0496) knots 0 0 0 0 1 1 1 1
  spline S104 degree 3 poles (2.7696, -8.0496) (2.9722, -8.0496) (3.1387, -7.8919) (3.1502, -7.6919) knots 0 0 0 0 1 1 1 1
  spline S105 degree 3 poles (3.1502, -0.4858) (3.1519, -0.4796) (3.1519, -0.4717) (3.1519, -0.462) knots 0 0 0 0 1 1 1 1
  spline S106 degree 3 poles (3.1519, -0.462) (3.1519, -0.2523) (2.981, -0.0805) (2.7696, -0.0805) knots 0 0 0 0 1 1 1 1
  spline S107 degree 3 poles (2.7696, -0.0805) (2.5581, -0.0805) (2.3881, -0.2523) (2.3881, -0.462) knots 0 0 0 0 1 1 1 1
  spline S108 degree 3 poles (2.3881, -0.462) (2.3881, -0.6726) (2.5581, -0.8444) (2.7696, -0.8444) knots 0 0 0 0 1 1 1 1
  spline S109 degree 3 poles (2.7696, -0.8444) (2.9722, -0.8444) (3.1387, -0.6867) (3.1502, -0.4858) knots 0 0 0 0 1 1 1 1
extrude "Extrude1" add sketch "Sketch1" along normal blind 1
